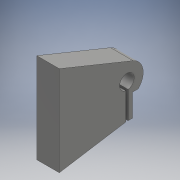
# Autodesk Inventor part: mocowanie walka
Saved by Autodesk Inventor 2017 (Build 210142000, 142)
## iProperties
Created: 2021-05-23
Part Number: mocowanie walka
Material: Generic
Document SubType Name: Modeling
Designer: majch
Density: 1 g/cm^3
Appearance: Smooth - Medium Gray
Author: majch
Autodesk Inventor part; units mm, degrees
ref_plane "YZ Plane" through (0, 0, 0) normal (1, 0, 0) x (0, 1, 0)
ref_plane "XZ Plane" through (0, 0, 0) normal (0, 1, 0) x (-1, 0, 0)
ref_plane "XY Plane" through (0, 0, 0) normal (0, 0, 1) x (1, 0, 0)
sketch "Sketch1" plane through (0, 0, 0) normal (1, 0, 0) x (0, 1, 0)
  arc A0 (30.5, -3.2113) -> (29.5, -3.2113) centre (30, 0) ccw
  arc A1 (35, -5.25) -> (32.7265, 6.7178) centre (30, 0) ccw
  line L0 (0, 0) -> (50.3094, 0) construction
  line L1 (0, 20) -> (0, -20)
  line L2 (0, 20) -> (32.7265, 6.7178)
  line L3 (30, 0) -> (30, -135) construction
  line L4 (30.5, -3.2113) -> (30.5, -15.25)
  line L5 (32.5, -5.25) -> (32.5, -15.25)
  line L6 (32.5, -5.25) -> (35, -5.25)
  line L7 (32.5, -15.25) -> (30.5, -15.25)
  line L8 (29.5, -3.2113) -> (29.5, -15.25)
  line L9 (0, -20) -> (29.5, -15.25)
  point P0 (30, -3.25)
  dimension "d1" = 6.5
  dimension "d2" = 30
  dimension "d3" = 14.5
  dimension "d4" = 40
  dimension "d17" = 0.5
  dimension "d18" = 10
  dimension "d19" = 2
  dimension "d20" = 2
  dimension "d21" = 1
  dimension "d24" = 20
  constraints: 20 end point, 4 point on circle, 3 horizontal, 3 vertical, 2 centre point, 2 point on line, 1 coincident, 1 midpoint, 1 parallel, 1 tangent
  measures "d1" diameter of A0
  measures "d2" distance of L0.start A0.centre
  measures "d3" diameter of A1
  measures "d4" distance of L1.start L1.end
  measures "d17" distance between parallel lines of L3 L4
  measures "d18" distance of L5.start L5.end
  measures "d19" vertical distance of point (30, -3.25) L5.start
  measures "d20" distance between parallel lines of L4 L5
  measures "d21" distance between parallel lines of L8 L4
  measures "d24" distance of L1.end L0.start
extrude "Extrusion1" add sketch "Sketch1" along normal blind 10
sketch "Sketch2" plane through (0, 32.5, -5.25) normal (0, 1, 0) x (1, 0, 0)
  line L0 (5, -5.25) -> (5, 25.2229) construction
  line L1 (0, 10) -> (0, 0) construction
  arc A0 (2.75, 4.25) -> (7.25, 4.25) centre (5, 4.25) ccw
  arc A1 (7.25, 5.75) -> (2.75, 5.75) centre (5, 5.75) ccw
  line L2 (2.75, 4.25) -> (2.75, 5.75)
  line L3 (7.25, 4.25) -> (7.25, 5.75)
  line L4 (0, 10) -> (10, 10) projected
  line L5 (0, 10) -> (0, 0) projected
  line L6 (0, 0) -> (10, 0) projected
  line L7 (10, 10) -> (10, 0) projected
  line L8 (0, 10) -> (10, 10) projected
  point P0 (0, -5.25)
  dimension "d27" = 5
  dimension "d28" = 4.5
  dimension "d29" = 4.5
  dimension "d30" = 1.5
  dimension "d31" = 4.25
  constraints: 6 end point, 4 point on circle, 3 tangent, 2 centre point, 2 point on line, 2 vertical
  measures "d27" distance between parallel lines of L1 L0
  measures "d28" diameter of A0
  measures "d29" diameter of A1
  measures "d30" distance of A1.centre A0.centre
  measures "d31" distance from line of A1.centre L4
extrude "Extrusion2" cut sketch "Sketch2" against normal up to surface (2 mm away) contours L2 A1 L3 A0
sketch "Sketch3" plane through (0, 29.5, -3.2113) normal (0, 1, 0) x (1, 0, 0)
  line L0 (2.75, 6.2887) -> (2.75, 7.7887) projected
  arc A0 (7.25, 7.7887) -> (2.75, 7.7887) centre (5, 7.7887) ccw projected
  line L1 (7.25, 7.7887) -> (7.25, 6.2887) projected
  arc A1 (2.75, 6.2887) -> (7.25, 6.2887) centre (5, 6.2887) ccw projected
  line L2 (0, 12.0387) -> (0, 2.0387) projected
  line L3 (0, 2.0387) -> (10, 2.0387) projected
  line L4 (10, 12.0387) -> (10, 2.0387) projected
  line L5 (0, 12.0387) -> (10, 12.0387) projected
  circle A2 centre (5, 7.0387) radius 2
  line L6 (5, 6.2887) -> (5, 7.7887)
  point P0 (0, -3.2113)
  dimension "d34" = 4
  dimension "d35" = 1.5
  dimension "d36" = 0.75
  constraints: 2 coincident, 2 end point, 1 centre point, 1 midpoint
  measures "d34" diameter of A2
  measures "d35" distance of L6.start L6.end
  measures "d36" distance of A0.centre A2.centre
extrude "Extrusion3" cut sketch "Sketch3" against normal blind 10 contours A2
equation "\"d17\" = 0.5 * d21"
equation "\"d24\" = 0.5 * d4"
equation "\"d36\" = 0.5 * d35"
body "Solid1"
